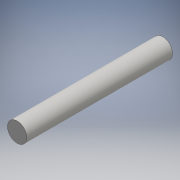
# Autodesk Inventor part: poal1
Saved by Autodesk Inventor 2016 SP1 (Build 200210100, 210)
## iProperties
Created: 2017-01-24
Part Number: poal1
Material: 一般
Document SubType Name: Modeling
Designer: p_admin
Density: 1 g/cm^3
Appearance: 既定
Author: p_admin
Autodesk Inventor part; units mm, degrees
ref_plane "YZ Plane" through (0, 0, 0) normal (1, 0, 0) x (0, 1, 0)
ref_plane "XZ Plane" through (0, 0, 0) normal (0, 1, 0) x (-1, 0, 0)
ref_plane "XY Plane" through (0, 0, 0) normal (0, 0, 1) x (1, 0, 0)
sketch "スケッチ1" plane through (0, 0, 0) normal (0, 1, 0) x (-1, 0, 0)
  circle A0 centre (0, 0) radius 100
  dimension "d0" = 200
  constraints: 1 centre point, 1 coincident
  measures "d0" diameter of A0
extrude "押し出し1" add sketch "スケッチ1" along normal blind 1500
sketch "スケッチ2" plane through (0, 1500, 0) normal (0, 1, 0) x (1, 0, 0)
  circle A0 centre (0, 0) radius 25
  dimension "d3" = 50
  constraints: 1 centre point, 1 coincident
  measures "d3" diameter of A0
extrude "押し出し2" cut sketch "スケッチ2" against normal blind 50
sketch "スケッチ3" plane through (0, 1500, 0) normal (0, 1, 0) x (1, 0, 0)
  point P0 (0, 0)
sketch "スケッチ4" plane through (0, 1500, 0) normal (0, 1, 0) x (1, 0, 0)
  circle A0 centre (0, 0) radius 25 projected
  circle A1 centre (0, 0) radius 50
  dimension "d6" = 100
  constraints: 1 centre point, 1 coincident
  measures "d6" diameter of A1
extrude "押し出し3" cut sketch "スケッチ4" against normal blind 120 contours A0 | A1
sketch "スケッチ5" plane through (0, 1500, 0) normal (0, 1, 0) x (1, 0, 0)
  circle A0 centre (0, 0) radius 52.5
  dimension "d9" = 105
  constraints: 1 centre point, 1 coincident
  measures "d9" diameter of A0
extrude "押し出し4" cut sketch "スケッチ5" against normal blind 120
sketch "スケッチ6" plane through (0, 1380, 0) normal (0, 1, 0) x (1, 0, 0)
  circle A0 centre (0, 0) radius 52.5 projected
  arc A1 (0.3926, 52.4985) -> (-0.3135, -52.4991) centre (0, 0) ccw
  line L0 (-0.3135, -52.4991) -> (0.3926, 52.4985)
  constraints: 4 point on circle, 2 end point, 1 centre point, 1 coincident
extrude "押し出し5" add sketch "スケッチ6" along normal blind 70 contours L0 A0 picked at (-3.2934, -17.1824)
